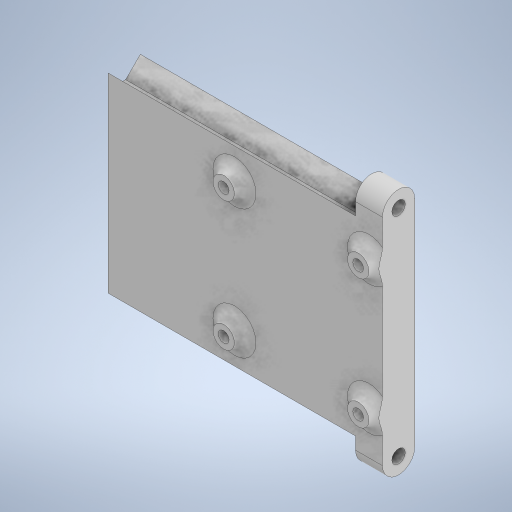
# Autodesk Inventor part: 카메라 홀더
Saved by Autodesk Inventor 2023 (Build 270158000, 158)
## iProperties
Created: 2022-11-10
Part Number: 카메라 홀더
Material: 일반
Document SubType Name: Modeling
Designer: user
Density: 1 g/cm^3
Appearance: 기본값
Author: user
Autodesk Inventor part; units mm, degrees
ref_plane "YZ Plane" through (0, 0, 0) normal (1, 0, 0) x (0, 1, 0)
ref_plane "XZ Plane" through (0, 0, 0) normal (0, 1, 0) x (-1, 0, 0)
ref_plane "XY Plane" through (0, 0, 0) normal (0, 0, 1) x (1, 0, 0)
sketch "스케치1" plane through (0, 0, 0) normal (0, 0, 1) x (1, 0, 0)
  line L0 (-25.5, 15) -> (25.5, 15)
  line L1 (25.5, 15) -> (25.5, -15)
  line L2 (25.5, -15) -> (-25.5, -15)
  line L3 (-25.5, -15) -> (-25.5, 15)
  line L4 (-25.5, 15) -> (25.5, -15) construction
  line L5 (25.5, 15) -> (-25.5, -15) construction
  line L6 (-2, -12) -> (23, -12) construction
  line L7 (23, -12) -> (23, 12) construction
  line L8 (23, 12) -> (-2, 12) construction
  line L9 (-2, 12) -> (-2, -12) construction
  line L10 (-2, -12) -> (23, 12) construction
  line L11 (23, -12) -> (-2, 12) construction
  circle A0 centre (-2, 12) radius 1
  line L12 (10.5, 0) -> (13.8415, 0)
  line L13 (10.5, 0) -> (10.5, -2.9401)
  circle A1 centre (23, 12) radius 1
  circle A2 centre (-2, -12) radius 1
  circle A3 centre (23, -12) radius 1
  point P0 (0, 0)
  dimension "d0" = 51
  dimension "d1" = 30
  dimension "d2" = 2
  dimension "d3" = 15
  dimension "d4" = 24
  dimension "d5" = 25
  constraints: 28 end point, 4 centre point, 4 midpoint, 4 parallel, 3 horizontal, 3 perpendicular, 3 symmetric about line, 1 coincident, 1 horizontal alignment, 3 other
  measures "d0" distance of L0.start L0.end
  measures "d1" distance of L0.end L1.end
  measures "d2" diameter of A0
  measures "d3" distance from line of L1 L12.start
  measures "d4" distance of L6.end L7.end
  measures "d5" distance of L7.end L8.end
extrude "돌출1" add sketch "스케치1" along normal mid plane 6
sketch "스케치4" plane through (25.5, -15, -3) normal (1, 0, 0) x (0, 0, -1)
  line L0 (-6, -3) -> (0, -3)
  line L1 (0, -3) -> (0, 33)
  line L2 (0, 33) -> (-6, 33)
  line L3 (-6, 33) -> (-6, -3)
  line L4 (-6, -3) -> (0, 33) construction
  line L5 (0, -3) -> (-6, 33) construction
  line L6 (-6, 33) -> (-3, 30)
  line L7 (-3, 30) -> (0, 33)
  line L8 (0.1414, 32.8586) -> (-3, 29.7172)
  line L9 (-3, 29.7172) -> (-6, 32.7172)
  line L10 (-3, 15) -> (-1.4715, 15)
  line L11 (0.1414, -2.8586) -> (-3, 0.2828)
  line L12 (-3, 0.2828) -> (-6, -2.7172)
  line L13 (0, 30) -> (-6, 30) projected
  line L14 (-6, 0) -> (-6, 30) projected
  line L15 (0, 0) -> (-6, 0) projected
  line L16 (0, 30) -> (0, 0) projected
  point P0 (-6, 0)
  point P1 (0, -2.7172)
  point P2 (-6, 30)
  point P3 (0, 32.7172)
  point P4 (-5, 32.7172)
  point P5 (-2.7172, 0)
  point P6 (-3.2828, 0)
  point P7 (-3.2828, 30)
  point P8 (-2.7172, 30)
  dimension "d25" = 36
  dimension "d27" = 90
  dimension "d28" = 0.2
  constraints: 26 end point, 3 symmetric about line, 2 horizontal, 2 midpoint, 2 parallel, 2 point on line, 1 perpendicular, 1 vertical alignment, 1 other
  measures "d25" distance of L0.end L1.end
  measures "d27" angle of L7 L6
  measures "d28" distance between parallel lines of L7 L8
extrude "돌출3" add sketch "스케치4" against normal up to surface (51 mm away) contours L3 L15 L12 | L11 L15 L1 | L3 L9 L13 | L13 L8 L1
sketch "스케치6" plane through (25.5, -17.7172, 3) normal (1, 0, 0) x (0, 0, -1)
  circle A0 centre (3, 37.7172) radius 3
  circle A1 centre (3, 37.7172) radius 1.25
  line L0 (3, 17.7172) -> (21.0559, 17.7172)
  circle A2 centre (3, -2.2828) radius 3
  circle A3 centre (3, -2.2828) radius 1.25
  line L1 (0, 35.4343) -> (0, 0) projected
  line L2 (0, 35.4343) -> (0, 37.7172)
  line L3 (6, 0) -> (6, 35.4343) projected
  line L4 (6, 37.7172) -> (6, 35.4343)
  line L5 (0, -2.2828) -> (0, 0)
  line L6 (6, -2.2828) -> (6, 0)
  line L7 (3.2828, 32.7172) -> (2.7172, 32.7172) projected
  line L8 (2.7172, 32.7172) -> (0, 35.4343) projected
  line L9 (0, 35.4343) -> (0, 0) projected
  line L10 (0, 0) -> (2.7172, 2.7172) projected
  line L11 (3.2828, 2.7172) -> (2.7172, 2.7172) projected
  line L12 (3.2828, 2.7172) -> (6, 0) projected
  line L13 (6, 0) -> (6, 35.4343) projected
  line L14 (6, 35.4343) -> (3.2828, 32.7172) projected
  dimension "d36" = 6
  dimension "d37" = 2.5
  dimension "d38" = 40
  constraints: 10 end point, 4 centre point, 4 point on circle, 2 coincident, 2 symmetric about line, 2 tangent, 2 vertical, 1 horizontal, 1 vertical alignment, 2 other
  measures "d36" diameter of A0
  measures "d37" diameter of A1
  measures "d38" distance of A2.centre A0.centre
extrude "돌출5" add sketch "스케치6" against normal blind 5 contours A0 | L4 L14 L7 L8 L2 A0 | L10 L11 L12 L6 A2 L5 | A2
sketch "스케치7" plane through (0, 0, 3) normal (0, 0, 1) x (1, 0, 0)
  circle A0 centre (-2, 12) radius 1 projected
  circle A1 centre (-2, 12) radius 2
  circle A2 centre (23, 12) radius 1 projected
  circle A3 centre (23, 12) radius 2
  circle A4 centre (-2, -12) radius 1 projected
  circle A5 centre (-2, -12) radius 2
  circle A6 centre (23, -12) radius 1 projected
  circle A7 centre (23, -12) radius 2
  point P0 (0, 0)
  dimension "d41" = 4
  dimension "d42" = 4
  dimension "d43" = 4
  dimension "d44" = 4
  constraints: 4 centre point, 4 coincident
  measures "d41" diameter of A1
  measures "d42" diameter of A3
  measures "d43" diameter of A5
  measures "d44" diameter of A7
extrude "돌출6" add sketch "스케치7" along normal blind 2
fillet "모깎기1" radius 2 4 edges at (-4, 12, 3) (21, 12, 3) (-4, -12, 3) (21, -12, 3)
